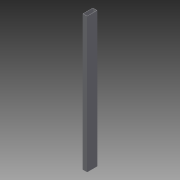
# Autodesk Inventor part: squareTube1.75x4
Saved by Autodesk Inventor 2014 (Build 180170000, 170)
## iProperties
Created: 2012-10-22
Part Number: squareTube1.75x4
Material: Generic
Document SubType Name: Modeling
Designer: istvan.burbank
Density: 1 g/cm^3
Appearance: Default
Author: istvan.burbank
Autodesk Inventor part; units mm, degrees
ref_plane "YZ Plane" through (0, 0, 0) normal (1, 0, 0) x (0, 1, 0)
ref_plane "XZ Plane" through (0, 0, 0) normal (0, 1, 0) x (-1, 0, 0)
ref_plane "XY Plane" through (0, 0, 0) normal (0, 0, 1) x (1, 0, 0)
sketch "Sketch1" plane through (0, 0, 0) normal (0, 1, 0) x (-1, 0, 0)
  line L0 (0, 0) -> (44.45, 0)
  line L1 (44.45, 0) -> (44.45, -101.6)
  line L2 (44.45, -101.6) -> (0, -101.6)
  line L3 (0, -101.6) -> (0, 0)
  line L4 (3.175, -98.425) -> (41.275, -98.425)
  line L5 (41.275, -98.425) -> (41.275, -3.175)
  line L6 (41.275, -3.175) -> (3.175, -3.175)
  line L7 (3.175, -3.175) -> (3.175, -98.425)
  dimension "d0" = 44.45
  dimension "d1" = 101.6
  dimension "d2" = 3.175
  constraints: 16 end point, 4 parallel, 2 perpendicular, 1 horizontal, 3 other
  measures "d0" distance of L1.end L2.end
  measures "d1" distance of L0.end L1.end
  measures "d2" distance between parallel lines of L3 L7
extrude "Extrusion1" add sketch "Sketch1" along normal blind 1346.2
body "Solid1"
